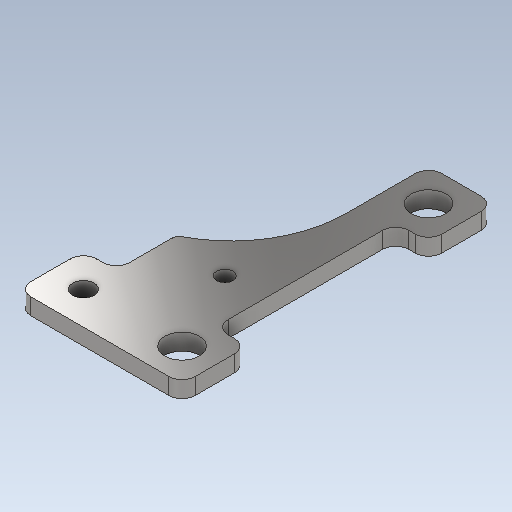
# Autodesk Inventor part: Side
Saved by Autodesk Inventor 2021 (Build 250183000, 183)
## iProperties
Created: 2021-02-06
Part Number: Side
Material: Steel, Mild
Document SubType Name: Modeling
Designer: buntykrgdg
Density: 7.85 g/cm^3
Appearance: Semi-Polished
Author: buntykrgdg
Autodesk Inventor part; units mm, degrees
ref_plane "YZ Plane" through (0, 0, 0) normal (1, 0, 0) x (0, 1, 0)
ref_plane "XZ Plane" through (0, 0, 0) normal (0, 1, 0) x (-1, 0, 0)
ref_plane "XY Plane" through (0, 0, 0) normal (0, 0, 1) x (1, 0, 0)
sketch "Sketch1" plane through (0, 0, 0) normal (0, 1, 0) x (-1, 0, 0)
  line L0 (4, 0) -> (46, 0)
  line L1 (50, -4) -> (50, -16)
  line L2 (46, -20) -> (44, -20)
  line L3 (40, -24) -> (40, -37.0175)
  line L4 (4, -95) -> (16, -95)
  line L5 (20, -91) -> (20, -75)
  arc A0 (50, -4) -> (46, 0) centre (46, -4) ccw
  arc A1 (46, -20) -> (50, -16) centre (46, -16) ccw
  arc A2 (16, -95) -> (20, -91) centre (16, -91) ccw
  arc A3 (0, -91) -> (4, -95) centre (4, -91) ccw
  arc A4 (4, 0) -> (0, -4) centre (4, -4) ccw
  arc A5 (44, -20) -> (40, -24) centre (44, -24) ccw
  line L6 (4, -20) -> (6, -20)
  line L7 (10, -24) -> (10, -71)
  line L8 (6, -75) -> (4, -75)
  line L9 (0, -4) -> (0, -16)
  line L10 (0, -79) -> (0, -91)
  arc A6 (0, -16) -> (4, -20) centre (4, -16) ccw
  arc A7 (10, -24) -> (6, -20) centre (6, -24) ccw
  arc A8 (6, -75) -> (10, -71) centre (6, -71) ccw
  arc A9 (4, -75) -> (0, -79) centre (4, -79) ccw
  line L11 (20, -69.8808) -> (20, -75)
  arc A10 (38.9189, -38.7939) -> (20, -69.8808) centre (55, -69.8808) ccw
  arc A11 (38.9189, -38.7939) -> (40, -37.0175) centre (38, -37.0175) ccw
  point P0 (0, 0)
  point P1 (0, -95)
  point P2 (50, 0)
  point P3 (50, -20)
  point P4 (40, -20)
  point P5 (20, -95)
  point P6 (40, -38.258)
  point P7 (0, -20)
  point P8 (10, -20)
  point P9 (10, -75)
  point P10 (0, -75)
  dimension "d0" = 95
  dimension "d1" = 50
  dimension "d2" = 20
  dimension "d3" = 10
  dimension "d5" = 20
  dimension "d6" = 20
  dimension "d8" = 4
  dimension "d10" = 10
  dimension "d11" = 55
  dimension "d12" = 10
  dimension "d13" = 4
  dimension "d30" = 35
  dimension "d31" = 2
  constraints: 25 point on circle, 25 tangent, 24 end point, 19 point on line, 12 centre point, 8 equal radius, 4 perpendicular, 3 horizontal, 3 vertical, 1 collinear
  measures "d0" distance of point (0, 0) point (0, -95)
  measures "d1" distance of point (0, 0) point (50, 0)
  measures "d2" distance of point (50, 0) point (50, -20)
  measures "d3" distance of point (50, -20) point (40, -20)
  measures "d5" distance of point (0, -95) point (20, -95)
  measures "d6" distance of point (20, -95) L5.end
  measures "d8" radius of A0
  measures "d10" distance of point (0, -20) point (10, -20)
  measures "d11" distance of point (10, -20) point (10, -75)
  measures "d12" distance of point (10, -75) point (0, -75)
  measures "d13" radius of A6
  measures "d30" radius of A10
  measures "d31" radius of A11
extrude "Extrusion1" add sketch "Sketch1" along normal blind 5
sketch "Sketch2" plane through (0, 5, 0) normal (0, 1, 0) x (1, 0, 0)
  circle A0 centre (-40, 10) radius 3.25
  line L0 (-50, 16) -> (-50, 4) projected
  line L1 (-46, 0) -> (-4, 0) projected
  circle A1 centre (-22, 35) radius 2.5
  line L2 (-10, 24) -> (-10, 71) projected
  circle A2 centre (-10, 10) radius 5.25
  line L3 (0, 4) -> (0, 16) projected
  circle A3 centre (-10, 85) radius 5.25
  line L4 (-4, 95) -> (-16, 95) projected
  line L5 (0, 79) -> (0, 91) projected
  point P0 (0, 0)
  dimension "d16" = 6.5
  dimension "d17" = 10
  dimension "d18" = 10
  dimension "d19" = 5
  dimension "d20" = 35
  dimension "d21" = 12
  dimension "d22" = 10.5
  dimension "d23" = 10
  dimension "d24" = 10
  dimension "d25" = 10.5
  dimension "d26" = 10
  dimension "d27" = 10
  constraints: 4 centre point
  measures "d16" diameter of A0
  measures "d17" distance from line of L0 A0.centre
  measures "d18" distance from line of A0.centre L1
  measures "d19" diameter of A1
  measures "d20" distance from line of A1.centre L1
  measures "d21" distance from line of A1.centre L2
  measures "d22" diameter of A2
  measures "d23" distance from line of L3 A2.centre
  measures "d24" distance from line of L1 A2.centre
  measures "d25" diameter of A3
  measures "d26" distance from line of L4 A3.centre
  measures "d27" distance from line of L5 A3.centre
extrude "Extrusion2" cut sketch "Sketch2" against normal through all
body "Solid1"
